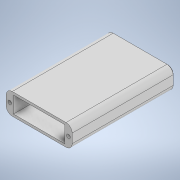
# Autodesk Inventor part: base
Saved by Autodesk Inventor 2021 (Build 250183000, 183)
## iProperties
Created: 2025-12-12
Part Number: base
Material: Generic
Document SubType Name: Modeling
Designer: Toby
Density: 1 g/cm^3
Appearance: Default
Author: Toby
Autodesk Inventor part; units mm, degrees
ref_plane "YZ Plane" through (0, 0, 0) normal (1, 0, 0) x (0, 1, 0)
ref_plane "XZ Plane" through (0, 0, 0) normal (0, 1, 0) x (-1, 0, 0)
ref_plane "XY Plane" through (0, 0, 0) normal (0, 0, 1) x (1, 0, 0)
sketch "Sketch1" plane through (0, 0, 0) normal (0, 0, 1) x (1, 0, 0)
  point P0 (0, 0)
sketch "Sketch2" plane through (0, 0, 0) normal (0, 0, 1) x (1, 0, 0)
  line L0 (-21, 6.75) -> (21, 6.75)
  line L1 (21, 6.75) -> (21, -6.75)
  line L2 (21, -6.75) -> (-21, -6.75)
  line L3 (-21, -6.75) -> (-21, 6.75)
  line L4 (-27, 8.75) -> (27, 8.75)
  line L5 (27, 8.75) -> (27, -8.75)
  line L6 (27, -8.75) -> (-27, -8.75)
  line L7 (-27, -8.75) -> (-27, 8.75)
  point P0 (0, 0)
  dimension "d0" = 42
  dimension "d1" = 13.5
  dimension "d2" = 2
  dimension "d3" = 2
  dimension "d4" = 6
  dimension "d5" = 6
  dimension "d6" = 6.75
  dimension "d7" = 21
  constraints: 16 end point, 4 parallel, 2 horizontal, 2 perpendicular
  measures "d0" distance of L0.start L0.end
  measures "d1" distance between parallel lines of L2 L0
  measures "d2" distance between parallel lines of L0 L4
  measures "d3" distance between parallel lines of L6 L2
  measures "d4" distance between parallel lines of L7 L3
  measures "d5" distance between parallel lines of L5 L1
  measures "d6" distance from line of point (0, 0) L0
  measures "d7" distance from line of point (0, 0) L3
extrude "Extrusion1" add sketch "Sketch2" along normal blind 82
sketch "Sketch3" plane through (0, 0, 0) normal (0, 0, -1) x (-1, 0, 0)
  line L0 (-27, -8.75) -> (-27, 8.75) projected
  line L1 (27, 8.75) -> (27, -8.75) projected
  line L2 (-27, 8.75) -> (27, 8.75)
  line L3 (27, 8.75) -> (27, -8.75)
  line L4 (27, -8.75) -> (-27, -8.75)
  line L5 (-27, -8.75) -> (-27, 8.75)
  point P0 (0, 0)
  constraints: 8 end point, 2 parallel, 1 horizontal, 1 perpendicular
extrude "Extrusion2" add sketch "Sketch3" along normal blind 1.2
fillet "Fillet1" radius 5 4 edges at (-27, 8.75, 40.4) (-27, -8.75, 40.4) (27, 8.75, 40.4) (27, -8.75, 40.4)
sketch "Sketch4" plane through (0, 0, 82) normal (0, 0, 1) x (1, 0, 0)
  line L0 (-21, -6.75) -> (-21, 6.75) projected
  line L1 (21, 6.75) -> (21, -6.75) projected
  line L2 (21, -6.75) -> (-21, -6.75) projected
  point P0 (0, 0)
  point P1 (-24, 0)
  point P2 (24, 0)
  dimension "d13" = 3
  dimension "d14" = 3
  dimension "d15" = 6.75
  dimension "d16" = 6.75
  measures "d13" distance from line of L0 point (-24, 0)
  measures "d14" distance from line of L1 point (24, 0)
  measures "d15" distance from line of L2 point (-24, 0)
  measures "d16" distance from line of L2 point (24, 0)
hole "Hole1" at (-24, 0, 82) at (24, 0, 82) direction (0, 0, -1) diameter 3 depth 8.8 tip angle 118
sketch "Sketch5" plane through (0, 0, 0) normal (0, 0, 1) x (1, 0, 0)
  line L0 (7.5, -1.05) -> (16.7, -1.05)
  line L1 (16.7, -1.05) -> (16.7, -4.55)
  line L2 (16.7, -4.55) -> (7.5, -4.55)
  line L3 (7.5, -4.55) -> (7.5, -1.05)
  line L4 (21, -6.75) -> (-21, -6.75) projected
  line L5 (21, 6.75) -> (21, -6.75) projected
  point P0 (0, 0)
  dimension "d24" = 2.2
  dimension "d25" = 3.5
  dimension "d26" = 9.2
  dimension "d27" = 4.3
  constraints: 8 end point, 2 parallel, 1 horizontal, 1 perpendicular
  measures "d24" distance between parallel lines of L4 L2
  measures "d25" distance between parallel lines of L2 L0
  measures "d26" distance of L0.start L0.end
  measures "d27" distance between parallel lines of L5 L1
extrude "Extrusion3" cut sketch "Sketch5" against normal blind 1.2
fillet "Fillet2" radius 1 4 edges at (16.7, -1.05, -0.6) (16.7, -4.55, -0.6) (7.5, -4.55, -0.6) (7.5, -1.05, -0.6)
sketch "Sketch6" plane through (0, 0, 0) normal (0, 0, 1) x (1, 0, 0)
  circle A0 centre (18.8, -2.8) radius 0.75
  line L0 (21, 6.75) -> (21, -6.75) projected
  line L1 (15.7, -4.55) -> (8.5, -4.55) projected
  line L2 (8.5, -1.05) -> (15.7, -1.05) projected
  point P0 (0, 0)
  dimension "d31" = 1.5
  dimension "d32" = 2.2
  dimension "d33" = 1.75
  dimension "d34" = 1.75
  constraints: 1 centre point
  measures "d31" diameter of A0
  measures "d32" distance from line of L0 A0.centre
  measures "d33" distance from line of L1 A0.centre
  measures "d34" distance from line of A0.centre L2
extrude "Extrusion4" cut sketch "Sketch6" against normal blind 1.2
chamfer "Chamfer1" distance 0.6 angle 45 8 edges at (12.1, -1.05, -1.2) (7.7929, -1.3429, -1.2) (7.5, -2.8, -1.2) (7.7929, -4.2571, -1.2) (12.1, -4.55, -1.2) (16.4071, -4.2571, -1.2) (16.7, -2.8, -1.2) (16.4071, -1.3429, -1.2)
chamfer "Chamfer2" distance 0.6 angle 45 8 edges at (0, 8.75, -1.2) (25.5355, 7.2855, -1.2) (27, 0, -1.2) (25.5355, -7.2855, -1.2) (0, -8.75, -1.2) (-25.5355, -7.2855, -1.2) (-27, 0, -1.2) (-25.5355, 7.2855, -1.2)
body "Solid1"
